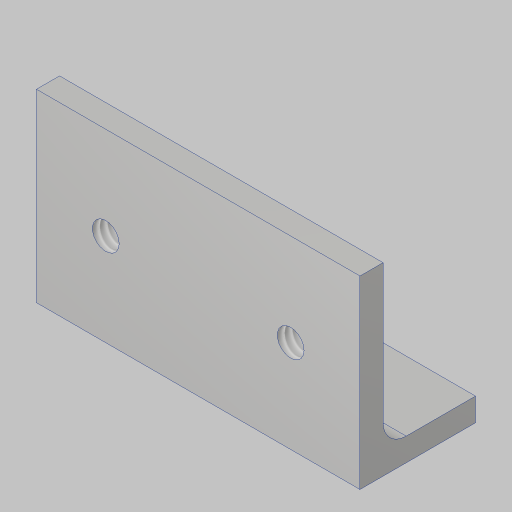
# Autodesk Inventor part: GP7-005
Saved by Autodesk Inventor 2023.5 (Build 275446000, 446)
## iProperties
Created: 2025-02-25
Part Number: GP7-005
Material: Aluminum 6061
Document SubType Name: Modeling
Designer: slick
Density: 2.7 g/cm^3
Appearance: Aluminum - Flat
Author: slick
Autodesk Inventor part; units mm, degrees
ref_plane "YZ Plane" through (0, 0, 0) normal (1, 0, 0) x (0, 1, 0)
ref_plane "XZ Plane" through (0, 0, 0) normal (0, 1, 0) x (-1, 0, 0)
ref_plane "XY Plane" through (0, 0, 0) normal (0, 0, 1) x (1, 0, 0)
sketch "Sketch1" plane through (0, 0, 0) normal (1, 0, 0) x (0, 1, 0)
  line L0 (0, 0) -> (25.4, 0)
  line L1 (25.4, 0) -> (25.4, -3.175)
  line L2 (25.4, -3.175) -> (3.175, -3.175)
  line L3 (3.175, -3.175) -> (3.175, -15.875)
  line L4 (3.175, -15.875) -> (0, -15.875)
  line L5 (0, -15.875) -> (0, 0)
  dimension "d0" = 25.4
  dimension "d2" = 3.175
  dimension "d21" = 15.875
  constraints: 12 end point, 6 perpendicular, 1 horizontal
  measures "d0" distance of L0.start L0.end
  measures "d2" distance between parallel lines of L5 L3
  measures "d21" distance of L4.end L0.start
extrude "Extrusion1" add sketch "Sketch1" along normal mid plane 44.45
fillet "Fillet1" radius 3.175 1 edges at (0, 3.175, -3.175)
sketch "Sketch2" plane through (-22.225, 0, -15.875) normal (0, -1, 0) x (1, 0, 0)
  line L0 (38.225, 9.525) -> (6.225, 9.525) construction
  line L1 (0, 15.875) -> (44.45, 15.875) construction
  point P0 (22.225, 15.875)
  point P1 (22.225, 9.525)
  point P2 (22.225, 15.875)
  dimension "d6" = 6.35
  dimension "d7" = 32
  constraints: 2 end point, 2 midpoint, 1 horizontal, 1 horizontal alignment, 1 vertical alignment
  measures "d6" distance between parallel lines of L1 L0
  measures "d7" distance of L0.start L0.end
hole "Hole1" at (16, 0, -6.35) at (-16, 0, -6.35) direction (0, 1, 0) diameter 2.6416 end through all thread size "6-32 UNC" class "2B" standard "ANSI Unified Screw Threads"
sketch "Sketch3" plane through (-22.225, 0, 0) normal (0, 0, 1) x (1, 0, 0)
  line L0 (0, 0) -> (44.45, 0) construction
  line L1 (0, 25.4) -> (44.45, 25.4) construction
  line L2 (34.925, 12.7) -> (9.525, 12.7) construction
  point P0 (22.225, 0)
  point P1 (22.225, 0)
  point P2 (22.225, 12.7)
  point P3 (22.225, 0)
  dimension "d15" = 25.4
  dimension "d22" = 12.7
  constraints: 3 midpoint, 2 end point, 1 horizontal, 1 horizontal alignment, 1 vertical alignment
  measures "d15" distance of L2.start L2.end
  measures "d22" distance between parallel lines of L2 L0
hole "Hole2" at (12.7, 12.7, 0) at (-12.7, 12.7, 0) direction (0, 0, -1) diameter 3.683 end through all thread size "10-24 UNC" class "2B" standard "ANSI Unified Screw Threads"
body "Solid1"
